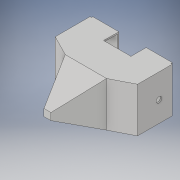
# Autodesk Inventor part: armorMk1
Saved by Autodesk Inventor 2019 (Build 230136000, 136)
## iProperties
Created: 2018-08-20
Part Number: armorMk1
Material: Generic
Document SubType Name: Modeling
Designer: Kitte_X
Density: 1 g/cm^3
Appearance: Default
Author: Kitte_X
Autodesk Inventor part; units mm, degrees
sketch "Sketch1" plane through (0, 0, 0) normal (0, 1, 0) x (-1, 0, 0)
  line L0 (65.8193, -27.9353) -> (65.8193, 275.5647)
  line L1 (65.8193, 275.5647) -> (634.8193, 275.5647)
  line L2 (634.8193, 275.5647) -> (634.8193, -27.9353)
  line L3 (448.3193, 71.0647) -> (252.3193, 71.0647)
  line L4 (448.3193, 71.0647) -> (448.3193, -27.9353)
  line L5 (252.3193, 71.0647) -> (252.3193, -27.9353)
  line L6 (65.8193, -27.9353) -> (252.3193, -27.9353)
  line L7 (448.3193, -27.9353) -> (634.8193, -27.9353)
  point P0 (0, 0)
  dimension "d0" = 569
  dimension "d1" = 303.5
  dimension "d2" = 196
  dimension "d3" = 186.5
  dimension "d4" = 99
  constraints: 16 end point, 4 perpendicular, 3 horizontal, 2 vertical
  measures "d0" distance of L0.start L2.end
  measures "d1" distance of L0.start L0.end
  measures "d2" distance of L3.start L3.end
  measures "d3" distance between parallel lines of L2 L4
  measures "d4" distance of L3.start L4.end
extrude "Extrusion1" add sketch "Sketch1" along normal blind 10
sketch "Sketch2" plane through (0, 0, 0) normal (0, -1, 0) x (1, 0, 0)
  line L0 (-65.8193, 275.5647) -> (-65.8193, -27.9353) projected
  line L1 (-65.8193, 275.5647) -> (-65.8193, -27.9353)
  line L2 (-65.8193, -27.9353) -> (-55.8193, -27.9353)
  line L3 (-55.8193, -27.9353) -> (-55.8193, 275.5647)
  line L4 (-55.8193, 275.5647) -> (-65.8193, 275.5647)
  line L5 (-634.8193, 275.5647) -> (-65.8193, 275.5647) projected
  line L6 (-634.8193, -27.9353) -> (-634.8193, 275.5647) projected
  line L7 (-634.8193, 275.5647) -> (-634.8193, -27.9353)
  line L8 (-634.8193, -27.9353) -> (-644.8193, -27.9353)
  line L9 (-644.8193, -27.9353) -> (-644.8193, 275.5647)
  line L10 (-644.8193, 275.5647) -> (-634.8193, 275.5647)
  point P0 (0, 0)
  dimension "d7" = 10
  dimension "d8" = 10
  constraints: 16 end point, 5 perpendicular, 2 point on line, 1 collinear, 1 vertical
  measures "d7" distance between parallel lines of L0 L3
  measures "d8" distance between parallel lines of L6 L9
extrude "Extrusion2" add sketch "Sketch2" along normal blind 300
extrude "Extrusion3" add sketch "Sketch2" against normal blind 10
sketch "Sketch3" plane through (0, 0, 0) normal (0, -1, 0) x (1, 0, 0)
  line L0 (-252.3193, -27.9353) -> (-65.8193, -27.9353) projected
  line L1 (-252.3193, -27.9353) -> (-65.8193, -27.9353)
  line L2 (-65.8193, -27.9353) -> (-65.8193, -37.9353)
  line L3 (-65.8193, -37.9353) -> (-252.3193, -37.9353)
  line L4 (-252.3193, -37.9353) -> (-252.3193, -27.9353)
  line L5 (-448.3193, 71.0647) -> (-448.3193, -27.9353) projected
  line L6 (-448.3193, -37.9353) -> (-448.3193, -27.9353)
  line L7 (-634.8193, -27.9353) -> (-634.8193, 275.5647) projected
  line L8 (-448.3193, -27.9353) -> (-634.8193, -27.9353)
  line L9 (-634.8193, -27.9353) -> (-634.8193, -37.9353)
  line L10 (-634.8193, -37.9353) -> (-448.3193, -37.9353)
  point P0 (0, 0)
  point P1 (-644.8193, -27.9353)
  point P2 (-541.5693, -37.9353)
  point P3 (-159.0693, -37.9353)
  point P4 (-448.3193, -32.9353)
  dimension "d13" = 10
  constraints: 16 end point, 6 perpendicular, 3 midpoint, 1 collinear, 1 horizontal alignment, 1 point on line
  measures "d13" distance of L0.end L2.end
extrude "Extrusion4" add sketch "Sketch3" against normal blind 10
extrude "Extrusion5" add sketch "Sketch3" along normal blind 300
ref_plane "Work Plane1" through (0, -150, 0) normal (0, -1, 0) x (1, 0, 0)
mirror "Mirror1" about plane through (0, -150, 0) normal (0, -1, 0) of "Extrusion1", "Extrusion4", "Extrusion3"
sketch "Sketch4" plane through (-644.8193, 10, -27.9353) normal (-1, 0, 0) x (0, 0, 1)
  circle A0 centre (95, -172.6482) radius 20
  line L0 (0, 0) -> (0, -320) projected
  point P0 (27.9353, -10)
  dimension "d20" = 40
  dimension "d21" = 95
  constraints: 1 centre point
  measures "d20" diameter of A0
  measures "d21" distance from line of L0 A0.centre
extrude "Extrusion6" cut sketch "Sketch4" against normal through all
sketch "Sketch5" plane through (0, 10, 0) normal (0, 1, 0) x (1, 0, 0)
  line L0 (-65.8193, -275.5647) -> (-634.8193, -275.5647) projected
  line L1 (-644.8193, 27.9353) -> (-644.8193, -275.5647) projected
  line L2 (-644.8193, -220.5647) -> (-519.8193, -220.5647)
  line L3 (-644.8193, -275.5647) -> (-55.8193, -275.5647) projected
  line L4 (-55.8193, -275.5647) -> (-55.8193, 27.9353) projected
  line L5 (-55.8193, -220.5647) -> (-55.8193, -275.5647)
  line L6 (-464.8193, -275.5647) -> (-55.8193, -275.5647)
  line L7 (-464.8193, -275.5647) -> (-644.8193, -275.5647)
  line L8 (-644.8193, -275.5647) -> (-644.8193, -220.5647)
  line L9 (-55.8193, -220.5647) -> (-519.8193, -220.5647)
  point P0 (0, 0)
  point P1 (-118.3193, -220.5647)
  point P2 (-582.3193, -220.5647)
  dimension "d27" = 125
  constraints: 12 end point, 4 point on line, 3 collinear, 2 horizontal, 1 horizontal alignment, 1 midpoint, 1 perpendicular
  measures "d27" distance of L2.start L2.end
extrude "Extrusion7" cut sketch "Sketch5" against normal through all
ref_plane "Work Plane3" through (-644.8193, 10, 570.5647) normal (0, 0, 1) x (1, 0, 0)
ref_plane "Work Plane4" through (-644.8193, 10, 295.5647) normal (0, 0, 1) x (1, 0, 0)
sketch "Sketch9" plane through (-644.8193, 10, 295.5647) normal (0, 0, 1) x (1, 0, 0)
  line L0 (146.5, -320) -> (146.5, 0)
  line L1 (146.5, 0) -> (442.5, 0)
  line L2 (442.5, 0) -> (442.5, -320)
  line L3 (442.5, -320) -> (146.5, -320)
  line L4 (10, -310) -> (579, -310) construction
  line L5 (392.5, -10) -> (392.5, -310) construction
  line L6 (579, -10) -> (10, -10) construction
  line L7 (0, 0) -> (589, 0) construction
  line L8 (156.5, -10) -> (156.5, -310) construction
  line L9 (156.5, -310) -> (432.5, -310) construction
  line L10 (432.5, -310) -> (432.5, -10) construction
  line L11 (432.5, -10) -> (156.5, -10) construction
  point P0 (644.8193, -10)
  point P1 (146.5, -160)
  point P2 (392.5, -160)
  point P3 (294.5, -10)
  point P4 (294.5, 0)
  point P5 (294.5, 0)
  point P6 (294.5, -320)
  dimension "d50" = 296
  dimension "d51" = 10
  constraints: 18 end point, 6 midpoint, 4 perpendicular, 1 coincident, 1 horizontal alignment, 1 vertical alignment, 3 other
  measures "d50" distance of L0.end L1.end
  measures "d51" distance between parallel lines of L0 L8
sketch "Sketch10" plane through (-644.8193, 10, 570.5647) normal (0, 0, 1) x (1, 0, 0)
  line L0 (269.5, -185) -> (319.5, -185)
  line L1 (319.5, -185) -> (319.5, -135)
  line L2 (319.5, -135) -> (269.5, -135)
  line L3 (269.5, -135) -> (269.5, -185)
  line L4 (196.5, -10) -> (196.5, -310) projected
  line L5 (579, -10) -> (10, -10) projected
  line L6 (279.5, -175) -> (279.5, -145) construction
  line L7 (279.5, -145) -> (309.5, -145) construction
  line L8 (309.5, -145) -> (309.5, -175) construction
  line L9 (309.5, -175) -> (279.5, -175) construction
  point P0 (644.8193, -10)
  point P1 (269.5, -160)
  point P2 (196.5, -160)
  point P3 (294.5, -135)
  point P4 (294.5, -10)
  dimension "d52" = 50
  dimension "d53" = 50
  dimension "d54" = 10
  constraints: 17 end point, 6 perpendicular, 4 midpoint, 1 horizontal, 1 horizontal alignment, 1 vertical alignment, 3 other
  measures "d52" distance of L2.end L0.start
  measures "d53" distance of L1.end L2.end
  measures "d54" distance between parallel lines of L3 L6
loft "Loft3" add profiles "Sketch9" section 1 edges at (-350.3193, -310, 220.5647) (-55.8193, -150, 220.5647) (-350.3193, 10, 220.5647) (-644.8193, -150, 220.5647)
sketch "Sketch11" plane through (-644.8193, 10, 295.5647) normal (0, 0, 1) x (1, 0, 0)
  line L0 (146.5, -320) -> (442.5, -320) construction
  line L1 (442.5, -320) -> (442.5, 0) construction
  line L2 (442.5, 0) -> (146.5, 0) construction
  line L3 (146.5, 0) -> (146.5, -320) construction
  line L4 (432.5, -10) -> (432.5, -310)
  line L5 (432.5, -310) -> (156.5, -310)
  line L6 (156.5, -310) -> (156.5, -10)
  line L7 (156.5, -10) -> (432.5, -10)
  point P0 (644.8193, -10)
  dimension "d59" = 10
  constraints: 8 end point, 3 other
  measures "d59" distance between parallel lines of L1 L4
loft "Loft4" cut profiles "Sketch11" section 1 edges at (-350.3193, -300, 220.5647) (-634.8193, -150, 220.5647) (-350.3193, 0, 220.5647) (-65.8193, -150, 220.5647)
loft "Loft5" add profiles "Sketch10" section 1 edges at (-350.3193, -310, 295.5647) (-202.3193, -150, 295.5647) (-350.3193, 10, 295.5647) (-498.3193, -150, 295.5647)
sketch "Sketch12" plane through (-644.8193, 10, 570.5647) normal (0, 0, 1) x (1, 0, 0)
  line L0 (309.5, -175) -> (309.5, -145)
  line L1 (309.5, -145) -> (279.5, -145)
  line L2 (279.5, -145) -> (279.5, -175)
  line L3 (279.5, -175) -> (309.5, -175)
  line L4 (319.5, -185) -> (269.5, -185) projected
  line L5 (319.5, -135) -> (319.5, -185) projected
  point P0 (644.8193, -10)
  point P1 (294.5, -175)
  point P2 (294.5, -185)
  point P3 (309.5, -160)
  point P4 (319.5, -160)
  dimension "d69" = 30
  dimension "d70" = 30
  constraints: 8 end point, 4 midpoint, 2 perpendicular, 1 horizontal alignment, 1 parallel, 1 vertical, 1 vertical alignment
  measures "d69" distance of L0.end L1.end
  measures "d70" distance of L1.end L2.end
loft "Loft6" cut profiles "Sketch12" section 1 edges at (-212.3193, -150, 295.5647) (-350.3193, -300, 295.5647) (-488.3193, -150, 295.5647) (-350.3193, 0, 295.5647)
extrude "Extrusion9" add sketch "Sketch10" against normal blind 10 draft 10
body "Solid1"
